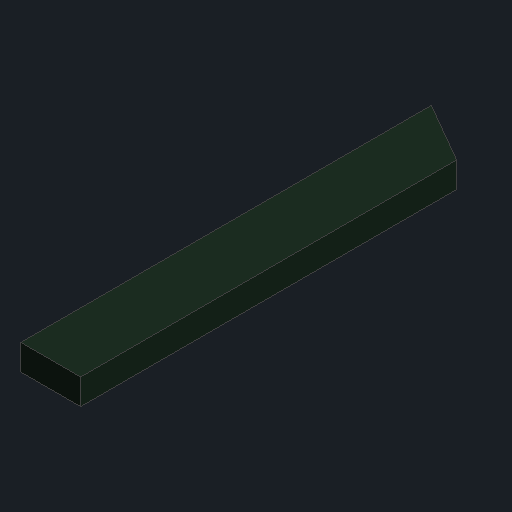
# Autodesk Inventor part: 2x4x24(with a cut)
Saved by Autodesk Inventor 2027 (Build 310192000, 192)
## iProperties
Created: 2026-05-29
Part Number: 2x4x24(with a cut)
Material: Generic
Document SubType Name: Modeling
Designer: lucas
Density: 1 g/cm^3
Appearance: Default
Author: lucas
Autodesk Inventor part; units mm, degrees
ref_plane "YZ Plane" through (0, 0, 0) normal (1, 0, 0) x (0, 1, 0)
ref_plane "XZ Plane" through (0, 0, 0) normal (0, 1, 0) x (-1, 0, 0)
ref_plane "XY Plane" through (0, 0, 0) normal (0, 0, 1) x (1, 0, 0)
sketch "Sketch1" plane through (0, 0, 0) normal (0, 1, 0) x (-1, 0, 0)
  line L0 (0, 0) -> (88.9, 0)
  line L1 (88.9, 0) -> (88.9, -609.6)
  line L2 (0, -558.2736) -> (88.9, -609.6)
  line L3 (0, 0) -> (0, -550.1386)
  line L4 (0, -550.1386) -> (0, -558.2736)
  point P0 (88.9, -550.1386)
  dimension "d2" = 609.6
  dimension "d6" = 88.9
  dimension "d7" = 60
  constraints: 10 end point, 3 vertical, 1 horizontal, 1 point on line
  measures "d2" distance of L0.end L1.end
  measures "d6" distance between parallel lines of L1 L3
  measures "d7" angle of L1 L2
extrude "Extrusion1" add sketch "Sketch1" along normal blind 38.1
body "Solid1"
